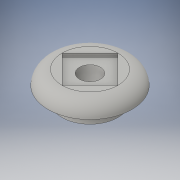
# Autodesk Inventor part: sleeve_support
Saved by Autodesk Inventor 2016 (Build 200138000, 138)
## iProperties
Created: 2016-02-05
Part Number: sleeve_support
Material: Generic
Document SubType Name: Modeling
Designer: Matt Ruffner
Density: 1 g/cm^3
Appearance: Default
Author: Matt Ruffner
Autodesk Inventor part; units mm, degrees
ref_plane "YZ Plane" through (0, 0, 0) normal (1, 0, 0) x (0, 1, 0)
ref_plane "XZ Plane" through (0, 0, 0) normal (0, 1, 0) x (-1, 0, 0)
ref_plane "XY Plane" through (0, 0, 0) normal (0, 0, 1) x (1, 0, 0)
sketch "Sketch2" plane through (0, 0, 0) normal (0, 0, 1) x (1, 0, 0)
  line L0 (0, 0) -> (19.05, 0)
  line L1 (19.05, 0) -> (19.05, 6.35)
  line L2 (12.7, 12.7) -> (0, 12.7)
  line L3 (0, 12.7) -> (0, 0)
  arc A0 (19.05, 6.35) -> (12.7, 12.7) centre (12.7, 6.35) ccw
  line L4 (19.05, 6.35) -> (12.7, 6.35)
  line L5 (12.7, 6.35) -> (12.7, 0)
  line L6 (4.7625, 0) -> (4.7625, -3.6847)
  line L7 (4.7625, -3.6847) -> (6.35, -3.6847)
  line L8 (6.35, -3.6847) -> (6.35, 0)
  dimension "d8" = 6.35
  dimension "d9" = 12.7
  dimension "d10" = 19.05
  dimension "d11" = 7.9375
  dimension "d12" = 1.5875
  constraints: 18 end point, 4 perpendicular, 3 point on line, 2 horizontal, 2 parallel, 2 point on circle, 2 tangent, 1 centre point, 1 vertical
  measures "d8" radius of A0
  measures "d9" distance of L2.end L0.start
  measures "d10" distance of L0.start L0.end
  measures "d11" distance between parallel lines of L5 L6
  measures "d12" distance of L6.end L7.end
revolve "Revolution1" add sketch "Sketch2" angle 360 about axis through (0, 12.7, 0) along (0, -1, 0) contours L3 L2 A0 L4 L5 L0 | L0 L8 L7 L6
sketch "Sketch3" plane through (0, 12.7, 0) normal (0, 1, 0) x (1, 0, 0)
  circle A0 centre (0, 0) radius 4.7625
  dimension "d14" = 9.525
  constraints: 1 centre point, 1 coincident
  measures "d14" diameter of A0
extrude "Extrusion1" cut sketch "Sketch3" against normal through all
sketch "Sketch4" plane through (0, 12.7, 0) normal (0, 1, 0) x (1, 0, 0)
  circle A0 centre (0, 0) radius 12.7 projected
  line L0 (-12.7, 0) -> (0, 12.7)
  line L1 (12.7, 0) -> (0, 12.7)
  line L2 (12.7, 0) -> (0, -12.7)
  line L3 (-12.7, 0) -> (0, -12.7)
  constraints: 8 end point, 5 point on circle, 3 perpendicular, 1 point on line
extrude "Extrusion2" cut sketch "Sketch4" against normal blind 1.5875 contours L2 L3 L0 L1
equation "\"d15\" = d14"
body "Solid1"
